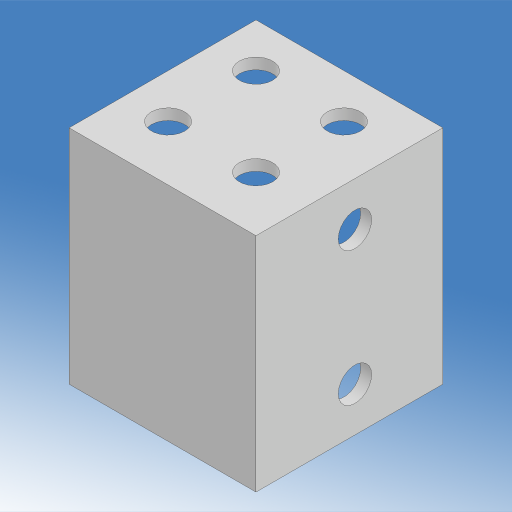
# Autodesk Inventor part: FlipperTensionerBlock2Tool
Saved by Autodesk Inventor 2024 (Build 280153000, 153)
## iProperties
Created: 2024-04-13
Part Number: FlipperTensionerBlock2Tool
Material: Generic
Document SubType Name: Modeling
Designer: seene
Density: 1 g/cm^3
Appearance: Default
Author: seene
Autodesk Inventor part; units mm, degrees
ref_plane "YZ Plane" through (0, 0, 0) normal (1, 0, 0) x (0, 1, 0)
ref_plane "XZ Plane" through (0, 0, 0) normal (0, 1, 0) x (-1, 0, 0)
ref_plane "XY Plane" through (0, 0, 0) normal (0, 0, 1) x (1, 0, 0)
sketch "Sketch1" plane through (0, 0, 0) normal (0, 1, 0) x (-1, 0, 0)
  line L0 (0, 0) -> (25.4, 0)
  line L1 (25.4, 0) -> (25.4, -25.4)
  line L2 (25.4, -25.4) -> (0, -25.4)
  line L3 (0, -25.4) -> (0, 0)
  line L4 (-1.5875, 1.5875) -> (26.9875, 1.5875)
  line L5 (26.9875, 1.5875) -> (26.9875, -26.9875)
  line L6 (26.9875, -26.9875) -> (-1.5875, -26.9875)
  line L7 (-1.5875, -26.9875) -> (-1.5875, 1.5875)
  circle A0 centre (19.05, -6.35) radius 2.413
  circle A1 centre (19.05, -19.05) radius 2.413
  circle A2 centre (6.35, -6.35) radius 2.413
  circle A3 centre (6.35, -19.05) radius 2.413
  dimension "d0" = 25.4
  dimension "d1" = 25.4
  dimension "d2" = 1.5875
  dimension "d3" = 6.35
  dimension "d4" = 6.35
  dimension "d5" = 4.826
  dimension "d8" = 12.7
  dimension "d11" = 12.7
  constraints: 16 end point, 4 centre point, 4 parallel, 2 horizontal, 2 perpendicular, 1 vertical, 9 other
  measures "d0" distance of L1.end L2.end
  measures "d1" distance of L0.end L1.end
  measures "d2" distance between parallel lines of L3 L7
  measures "d3" distance from line of A0.centre L1
  measures "d4" distance from line of L0 A0.centre
  measures "d5" diameter of A0
  measures "d8" distance of A0.centre A1.centre
  measures "d11" distance of A0.centre A2.centre
extrude "Extrusion1" add sketch "Sketch1" against normal blind 1.5875 contours L0 L1 L2 L3 | L4 L5 L6 L7
extrude "Extrusion2" add sketch "Sketch1" against normal blind 32.0675 contours L4 L5 L6 L7
sketch "Sketch2" plane through (1.5875, 0, 1.5875) normal (1, 0, 0) x (0, 0, -1)
  line L0 (0, 0) -> (28.575, 0) construction
  line L1 (14.2875, 0) -> (14.2875, -32.0675) construction
  line L2 (26.9875, -32.0675) -> (1.5875, -32.0675) construction
  circle A0 centre (14.2875, -6.35) radius 2.413
  circle A1 centre (14.2875, -25.7175) radius 2.413
  point P0 (1.5875, 0)
  dimension "d18" = 4.826
  dimension "d19" = 4.826
  dimension "d20" = 6.35
  dimension "d21" = 6.35
  constraints: 2 centre point, 2 end point, 2 midpoint, 2 point on line
  measures "d18" diameter of A0
  measures "d19" diameter of A1
  measures "d20" distance from line of L2 A1.centre
  measures "d21" distance from line of L0 A0.centre
extrude "Extrusion3" cut sketch "Sketch2" against normal blind 32.0675
sketch "Sketch3" plane through (-26.9875, 0, -26.9875) normal (-1, 0, 0) x (0, 0, 1)
  circle A0 centre (14.2875, -25.7175) radius 2.413 projected
  circle A1 centre (14.2875, -6.35) radius 2.413 projected
  line L0 (0, 0) -> (28.575, 0) projected
  line L1 (0, 0) -> (0, -32.0675) projected
  line L2 (28.575, -32.0675) -> (0, -32.0675) projected
  line L3 (28.575, 0) -> (28.575, -32.0675) projected
  point P0 (26.9875, 0)
sketch "Sketch4" plane through (1.5875, 0, -26.9875) normal (0, 0, -1) x (-1, 0, 0)
  line L0 (0, 0) -> (28.575, 0) projected
  line L1 (0, 0) -> (0, -32.0675) projected
  line L2 (28.575, -32.0675) -> (0, -32.0675) projected
  line L3 (28.575, 0) -> (28.575, -32.0675) projected
  point P0 (1.5875, 0)
extrude "Extrusion4" cut sketch "Sketch3" against normal blind 1.5875
extrude "Extrusion5" cut sketch "Sketch4" against normal blind 1.5875
equation "\"d18\" = d19"
equation "\"d21\" = d20"
body "Solid1"
